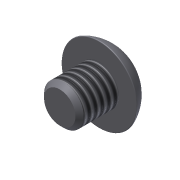
# Autodesk Inventor part: 10-32 BHCS x375
Saved by Autodesk Inventor 2013 (Build 170138000, 138)
## iProperties
Created: 2011-07-25
Part Number: 10-32 BHCS x375
Material: Steel
Document SubType Name: Modeling
Designer: Dan Niemitalo
Density: 7.85 g/cm^3
Author: Dan Niemitalo
Autodesk Inventor part; units mm, degrees
ref_plane "YZ Plane" through (0, 0, 0) normal (1, 0, 0) x (0, 1, 0)
ref_plane "XZ Plane" through (0, 0, 0) normal (0, 1, 0) x (-1, 0, 0)
ref_plane "XY Plane" through (0, 0, 0) normal (0, 0, 1) x (1, 0, 0)
sketch "Sketch1" plane through (0, 0, 0) normal (0, 0, 1) x (1, 0, 0)
  circle A0 centre (0, 0) radius 2.413
  dimension "d0" = 4.826
  constraints: 1 centre point, 1 coincident
  measures "d0" diameter of A0
extrude "Extrusion1" add sketch "Sketch1" along normal blind 4.7752
sketch "Sketch2" plane through (0, 0, 0) normal (0, 1, 0) x (-1, 0, 0)
  line L0 (0, 0) -> (0, -2.5654)
  line L1 (0, 0) -> (4.5085, 0)
  line L2 (0, -2.5654) -> (2.032, -2.5654)
  line L3 (4.5085, 0) -> (4.5085, 4.071) construction
  arc A0 (4.5791, -0.105) -> (4.5085, 0) centre (4.5085, -0.0762) ccw
  arc A1 (2.032, -2.5654) -> (4.5791, -0.105) centre (0.5168, 1.5517) ccw
  line L4 (4.5847, 0.6553) -> (4.5847, -0.0762) construction
  dimension "d3" = 2.5654
  dimension "d6" = 2.032
  dimension "d12" = 4.5847
  dimension "d18" = 0.0762
  constraints: 10 end point, 5 point on circle, 3 tangent, 2 centre point, 2 perpendicular, 1 horizontal, 1 parallel, 1 vertical
  measures "d3" distance of L0.start L0.end
  measures "d6" distance of L0.end L2.end
  measures "d12" distance between parallel lines of L0 L4
  measures "d18" radius of A0
revolve "Revolution1" add sketch "Sketch2" angle 360 about axis through (0, 0, 0) along (0, 0, -1)
sketch "Sketch3" plane through (0, 0, -2.5654) normal (0, 0, -1) x (-1, 0, 0)
  circle A0 centre (0, 0) radius 2.032 projected
  line L0 (-0.9165, 1.5875) -> (0.9165, 1.5875)
  line L1 (0.9165, 1.5875) -> (1.8331, 0)
  line L2 (1.8331, 0) -> (0.9165, -1.5875)
  line L3 (0.9165, -1.5875) -> (-0.9165, -1.5875)
  line L4 (-0.9165, -1.5875) -> (-1.8331, 0)
  line L5 (-1.8331, 0) -> (-0.9165, 1.5875)
  dimension "d8" = 3.175
  constraints: 12 end point, 1 coincident, 1 horizontal, 13 other
  measures "d8" distance between parallel lines of L3 L0
extrude "Extrusion2" cut sketch "Sketch3" against normal blind 1.5875 contours L0 L1 L2 L3 L4 L5
chamfer "Chamfer1" distance 0.508 angle 45 1 edges at (-2.413, 0, 4.7752)
thread "Thread1" size "10-32 UNF" class "2A" standard "ANSI Unified Screw Threads" full length
body "Solid1"
